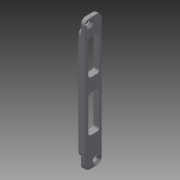
# Autodesk Inventor part: IOModulePlate01
Saved by Autodesk Inventor 2013 (Build 170138000, 138)
## iProperties
Created: 2014-07-14
Part Number: IOModulePlate01
Material: Generic
Document SubType Name: Modeling
Designer: spichelh
Density: 1 g/cm^3
Author: spichelh
Autodesk Inventor part; units mm, degrees
ref_plane "YZ Plane" through (0, 0, 0) normal (1, 0, 0) x (0, 1, 0)
ref_plane "XZ Plane" through (0, 0, 0) normal (0, 1, 0) x (-1, 0, 0)
ref_plane "XY Plane" through (0, 0, 0) normal (0, 0, 1) x (1, 0, 0)
sketch "Sketch1" plane through (0, 0, 0) normal (1, 0, 0) x (0, 1, 0)
  line L0 (2, 0) -> (50.8, 0)
  line L1 (52.8, -2) -> (52.8, -4.8)
  line L2 (50.8, -6.8) -> (2, -6.8)
  line L3 (0, -4.8) -> (0, -2)
  arc A0 (2, 0) -> (0, -2) centre (2, -2) ccw
  arc A1 (0, -4.8) -> (2, -6.8) centre (2, -4.8) ccw
  arc A2 (50.8, -6.8) -> (52.8, -4.8) centre (50.8, -4.8) ccw
  arc A3 (52.8, -2) -> (50.8, 0) centre (50.8, -2) ccw
  line L4 (26.4, 0) -> (26.4, -6.5481) construction
  line L5 (52.8, -3.4) -> (39.7965, -3.4) construction
  circle A4 centre (1.9, -4.9) radius 1
  circle A5 centre (50.9, -4.9) radius 1 construction
  circle A6 centre (50.9, -1.9) radius 1
  point P0 (0, 0)
  point P1 (52.8, 0)
  point P2 (0, -6.8)
  dimension "d0" = 52.8
  dimension "d1" = 6.8
  dimension "d2" = 2
  dimension "d19" = 2
  dimension "d20" = 0.1
  dimension "d21" = 0.1
  constraints: 12 end point, 8 point on circle, 8 tangent, 7 centre point, 6 point on line, 3 equal radius, 3 parallel, 2 midpoint, 2 perpendicular, 2 symmetric about line, 1 horizontal, 2 other
  measures "d0" distance of point (0, 0) point (52.8, 0)
  measures "d1" distance of point (0, -6.8) point (0, 0)
  measures "d2" radius of A0
  measures "d19" diameter of A4
  measures "d20" horizontal distance of A1.centre A4.centre
  measures "d21" horizontal distance of A1.centre A4.centre
extrude "Extrusion1" add sketch "Sketch1" along normal blind 1.5
chamfer "Chamfer1" distance 0.8 angle 45 2 edges at (1.5, 49.9, -1.9) (1.5, 0.9, -4.9)
sketch "Sketch2" plane through (1.5, 0, 0) normal (1, 0, 0) x (0, 0, -1)
  line L0 (0, 50.8) -> (0, 2) projected
  line L1 (2.5, 45.871) -> (4.9546, 45.871)
  line L2 (5.9546, 44.871) -> (5.9546, 32.8996)
  line L3 (4.9546, 31.8996) -> (2.5, 31.8996)
  line L4 (1.5, 32.8996) -> (1.5, 44.871)
  line L5 (2.5, 26.5) -> (4.9546, 26.5)
  line L6 (5.9546, 25.5) -> (5.9546, 12.7187)
  line L7 (4.9546, 11.7187) -> (2.5, 11.7187)
  line L8 (1.5, 12.7187) -> (1.5, 25.5)
  arc A0 (5.9546, 44.871) -> (4.9546, 45.871) centre (4.9546, 44.871) ccw
  arc A1 (2.5, 45.871) -> (1.5, 44.871) centre (2.5, 44.871) ccw
  arc A2 (1.5, 32.8996) -> (2.5, 31.8996) centre (2.5, 32.8996) ccw
  arc A3 (4.9546, 31.8996) -> (5.9546, 32.8996) centre (4.9546, 32.8996) ccw
  arc A4 (5.9546, 25.5) -> (4.9546, 26.5) centre (4.9546, 25.5) ccw
  arc A5 (4.9546, 11.7187) -> (5.9546, 12.7187) centre (4.9546, 12.7187) ccw
  arc A6 (1.5, 12.7187) -> (2.5, 11.7187) centre (2.5, 12.7187) ccw
  arc A7 (2.5, 26.5) -> (1.5, 25.5) centre (2.5, 25.5) ccw
  point P0 (0, 0)
  dimension "d9" = 1
  dimension "d10" = 1.5
  dimension "d11" = 1.5
  constraints: 16 end point, 16 point on circle, 16 tangent, 8 centre point, 7 equal radius, 4 parallel, 2 horizontal, 2 perpendicular
  measures "d9" radius of A0
  measures "d10" distance between parallel lines of L0 L4
  measures "d11" distance between parallel lines of L0 L8
extrude "Extrusion2" cut sketch "Sketch2" against normal blind 1.5
sketch "Sketch3" plane through (0, 0, 0) normal (-1, 0, 0) x (0, 0, 1)
  arc A0 (-1.5, 44.871) -> (-2.5, 45.871) centre (-2.5, 44.871) ccw projected
  line L0 (-1.5, 44.871) -> (-1.5, 32.8996) projected
  arc A1 (-2.5, 31.8996) -> (-1.5, 32.8996) centre (-2.5, 32.8996) ccw projected
  line L1 (-2.5, 31.8996) -> (-4.9546, 31.8996) projected
  arc A2 (-5.9546, 32.8996) -> (-4.9546, 31.8996) centre (-4.9546, 32.8996) ccw projected
  line L2 (-5.9546, 32.8996) -> (-5.9546, 44.871) projected
  arc A3 (-4.9546, 45.871) -> (-5.9546, 44.871) centre (-4.9546, 44.871) ccw projected
  line L3 (-4.9546, 45.871) -> (-2.5, 45.871) projected
  arc A4 (-4.9546, 26.5) -> (-5.9546, 25.5) centre (-4.9546, 25.5) ccw projected
  line L4 (-4.9546, 26.5) -> (-2.5, 26.5) projected
  arc A5 (-1.5, 25.5) -> (-2.5, 26.5) centre (-2.5, 25.5) ccw projected
  line L5 (-1.5, 25.5) -> (-1.5, 12.7187) projected
  arc A6 (-2.5, 11.7187) -> (-1.5, 12.7187) centre (-2.5, 12.7187) ccw projected
  line L6 (-2.5, 11.7187) -> (-4.9546, 11.7187) projected
  arc A7 (-5.9546, 12.7187) -> (-4.9546, 11.7187) centre (-4.9546, 12.7187) ccw projected
  line L7 (-5.9546, 12.7187) -> (-5.9546, 25.5) projected
  line L8 (0, 50.8) -> (0, 2) projected
  line L9 (-4.8, 52.8) -> (-2, 52.8) projected
  line L10 (-4.8, 48.8) -> (-2, 48.8)
  line L11 (0, 46.8) -> (0, 6)
  line L12 (-2, 4) -> (-4.8, 4)
  line L13 (-6.8, 6) -> (-6.8, 46.8)
  arc A8 (-4.8, 48.8) -> (-6.8, 46.8) centre (-4.8, 46.8) ccw
  arc A9 (0, 46.8) -> (-2, 48.8) centre (-2, 46.8) ccw
  arc A10 (-2, 4) -> (0, 6) centre (-2, 6) ccw
  arc A11 (-6.8, 6) -> (-4.8, 4) centre (-4.8, 6) ccw
  line L14 (-3.4, 52.8) -> (-3.4, 49.069) construction
  line L15 (-3.4, 48.8) -> (-3.4, 44.871) construction
  line L16 (0, 26.4) -> (-3, 26.4) construction
  line L17 (-6.8, 26.4) -> (-12.1303, 26.4) construction
  point P0 (0, 0)
  point P1 (0, 4)
  point P2 (0, 48.8)
  point P3 (-6.8, 4)
  point P4 (-6.8, 45.8508)
  point P5 (-6.8, 31.9198)
  point P6 (-6.8, 26.4798)
  point P7 (-6.8, 11.7389)
  dimension "d14" = 6.8
  dimension "d15" = 44.8
  dimension "d16" = 2
  constraints: 16 end point, 8 point on circle, 8 tangent, 6 point on line, 4 centre point, 4 collinear, 4 midpoint, 3 equal radius, 3 perpendicular, 2 parallel, 1 horizontal, 4 other
  measures "d14" distance of point (0, 4) point (-6.8, 4)
  measures "d15" distance of point (0, 48.8) point (0, 4)
  measures "d16" radius of A8
extrude "Extrusion3" add sketch "Sketch3" along normal blind 1
body "Solid1"
